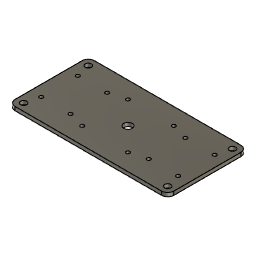
Platform_ bottom (Autodesk Fusion 360 design; units mm, degrees)
Autodesk Fusion 360 part; units mm, degrees
sketch "Sketch1" plane through (0, 0, 0) normal (0, 0, 1) x (1, 0, 0)
  line L0 (-60, 32.5) -> (0, 32.5)
  line L1 (0, -32.5) -> (-60, -32.5)
  line L2 (-65, -27.5) -> (-65, 27.5)
  arc A0 (-60, 32.5) -> (-65, 27.5) centre (-60, 27.5) ccw
  arc A1 (-65, -27.5) -> (-60, -32.5) centre (-60, -27.5) ccw
  circle A2 centre (-59, 26.5) radius 2.5
  circle A3 centre (-59, -26.5) radius 2.5
  circle A4 centre (0, 0) radius 3.5
  circle A5 centre (-56, 15) radius 1.5
  circle A6 centre (-56, -15) radius 1.5
  circle A7 centre (-32, 15) radius 1.5
  circle A8 centre (-32, -15) radius 1.5
  line L3 (0, 32.5) -> (0, -32.5) construction
  line L4 (65, -27.5) -> (65, 27.5)
  circle A9 centre (59, 26.5) radius 2.5
  arc A10 (60, -32.5) -> (65, -27.5) centre (60, -27.5) ccw
  circle A11 centre (32, 15) radius 1.5
  circle A12 centre (56, 15) radius 1.5
  circle A13 centre (56, -15) radius 1.5
  circle A14 centre (59, -26.5) radius 2.5
  arc A15 (65, 27.5) -> (60, 32.5) centre (60, 27.5) ccw
  line L5 (0, -32.5) -> (60, -32.5)
  line L6 (60, 32.5) -> (0, 32.5)
  circle A16 centre (32, -15) radius 1.5
  circle A17 centre (-18.75, 18.75) radius 1.5
  circle A18 centre (-18.75, -18.75) radius 1.5
  circle A19 centre (18.75, -18.75) radius 1.5
  circle A20 centre (18.75, 18.75) radius 1.5
  dimension "d1" = 65
  dimension "d3" = 32.5
  dimension "d4" = 32.5
  dimension "d5" = 5
  dimension "d6" = 5
  dimension "d9" = 5
  dimension "d10" = 6
  dimension "d11" = 6
  dimension "d12" = 5
  dimension "d13" = 6
  dimension "d14" = 6
  dimension "d21" = 7
  dimension "d24" = 9
  dimension "d25" = 9
  dimension "d26" = 30
  dimension "d27" = 3
  dimension "d28" = 3
  dimension "d29" = 17.5
  dimension "d30" = 3
  dimension "d31" = 3
  dimension "d32" = 30
  dimension "d33" = 17.5
  dimension "d34" = 24
  dimension "d35" = 65
  dimension "d36" = 65
  dimension "d41" = 3
  dimension "d42" = 3
  dimension "d43" = 37.5
  dimension "d44" = 13.75
  dimension "d45" = 18.75
  constraint horizontal L0
  constraint horizontal L1
  constraint vertical L2
  constraint tangent L0 A0
  constraint tangent L2 A0
  constraint tangent L1 A1
  constraint tangent L2 A1
  constraint coincident A4.centre origin
  constraint symmetric L0.start L3 A15.end
  constraint symmetric L2.end L3 L4.end
  constraint symmetric A0 L3 A15
  constraint symmetric L1.end L3 A10.start
  constraint symmetric L2.start L3 L4.start
  constraint symmetric A1 L3 A10
  constraint symmetric L0.end L3 L6.end
  constraint symmetric L1.start L3 L5.start
  constraint symmetric A2 L3 A9
  constraint symmetric A3 L3 A14
  constraint symmetric A5 L3 A12
  constraint symmetric A6 L3 A13
  constraint symmetric A7 L3 A11
  constraint symmetric A8 L3 A16
  constraint symmetric L3 A17 A20
  constraint symmetric L3 A18 A19
  measures "d1" distance of A4.centre L2
  measures "d3" distance of A4.centre L0
  measures "d4" distance of A4.centre L1
  measures "d5" radius of A0
  measures "d6" radius of A1
  measures "d9" diameter of A2
  measures "d10" distance of L0 A2.centre
  measures "d11" distance of L2 A2.centre
  measures "d12" diameter of A3
  measures "d13" distance of L1 A3.centre
  measures "d14" distance of L2 A3.centre
  measures "d21" diameter of A4
  measures "d24" distance of L2 A5.centre
  measures "d25" distance of L2 A6.centre
  measures "d26" distance of A5.centre A6.centre
  measures "d27" diameter of A5
  measures "d28" diameter of A6
  measures "d29" distance of L0 A5.centre
  measures "d30" diameter of A7
  measures "d31" diameter of A8
  measures "d32" distance of A7.centre A8.centre
  measures "d33" distance of L0 A7.centre
  measures "d34" distance of A5.centre A7.centre
  measures "d35" distance of L2 L0.end
  measures "d36" distance of L2 L1.start
  measures "d41" diameter of A17
  measures "d42" diameter of A18
  measures "d43" distance of A17.centre A18.centre
  measures "d44" distance of L0 A17.centre
  measures "d45" distance of L3 A18.centre
extrude "Extrude4" add sketch "Sketch1" along normal blind 3
equation "d3 = ( 65 / 2 ) * 1 mm"
equation "d4 = d3"
equation "d6 = d5"
equation "d11 = d10"
equation "d12 = d9"
equation "d13 = d10"
equation "d14 = d10"
equation "d25 = d24"
equation "d28 = d27"
equation "d30 = d27"
equation "d31 = d27"
equation "d32 = d26"
equation "d33 = d29"
equation "d35 = d1"
equation "d36 = d1"
equation "d42 = d41"
equation "d44 = d3 - d43 / 2"
equation "d45 = ( 37.5 / 2 ) * 1 mm"
